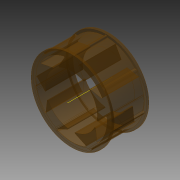
# Autodesk Inventor part: inner tread
Saved by Autodesk Inventor 2013 (Build 170138000, 138)
## iProperties
Created: 2013-05-09
Part Number: inner tread
Material: Generic
Document SubType Name: Modeling
Designer: grtstudent
Density: 1 g/cm^3
Author: grtstudent
Autodesk Inventor part; units mm, degrees
ref_plane "YZ Plane" through (0, 0, 0) normal (1, 0, 0) x (0, 1, 0)
ref_plane "XZ Plane" through (0, 0, 0) normal (0, 1, 0) x (-1, 0, 0)
ref_plane "XY Plane" through (0, 0, 0) normal (0, 0, 1) x (1, 0, 0)
sketch "Sketch1" plane through (0, 0, 0) normal (0, 0, 1) x (1, 0, 0)
  circle A0 centre (0, 0) radius 44.45
  circle A1 centre (11.1973, -15.4118) radius 1.905
  circle A2 centre (-18.1176, 5.8868) radius 1.905
  circle A3 centre (0, 19.05) radius 1.905
  circle A4 centre (-11.1973, -15.4118) radius 1.905
  circle A5 centre (18.1176, 5.8868) radius 1.905
  line L0 (-6.4158, 0) -> (-3.2079, 5.5563)
  line L1 (-3.2079, 5.5563) -> (3.2079, 5.5563)
  line L2 (3.2079, 5.5563) -> (6.4158, 0)
  line L3 (6.4158, 0) -> (3.2079, -5.5563)
  line L4 (3.2079, -5.5563) -> (-3.2079, -5.5563)
  line L5 (-3.2079, -5.5563) -> (-6.4158, 0)
  arc A6 (-6.9808, 33.2105) -> (-7.631, 34.0811) centre (-7.5009, 33.5002) ccw
  arc A7 (-7.631, 34.0811) -> (-30.055, 17.7891) centre (0, 0) ccw
  arc A8 (-30.055, 17.7891) -> (-29.4279, 16.9018) centre (-29.5427, 17.4859) ccw
  line L6 (-18.3896, 19.0716) -> (-29.4279, 16.9018)
  arc A9 (-17.8563, 18.0641) -> (-18.3896, 19.0716) centre (-18.2748, 18.4875) ccw
  arc A10 (-17.8563, 18.0641) -> (-25.0639, -4.1185) centre (0, 0) ccw
  arc A11 (-26.0876, -4.6201) -> (-25.0639, -4.1185) centre (-25.6513, -4.215) ccw
  line L7 (-33.7423, 3.6235) -> (-26.0876, -4.6201)
  arc A12 (-33.7423, 3.6235) -> (-34.7712, 3.2742) centre (-34.1785, 3.2184) ccw
  arc A13 (-34.7712, 3.2742) -> (-26.206, -23.0869) centre (0, 0) ccw
  arc A14 (-26.206, -23.0869) -> (-25.1682, -22.7646) centre (-25.7593, -22.6933) ccw
  line L8 (-23.8209, -11.5961) -> (-25.1682, -22.7646)
  arc A15 (-22.6979, -11.4002) -> (-23.8209, -11.5961) centre (-23.2299, -11.6674) ccw
  arc A16 (-22.6979, -11.4002) -> (-3.8282, -25.1098) centre (0, 0) ccw
  arc A17 (-3.6675, -26.2384) -> (-3.8282, -25.1098) centre (-3.918, -25.6984) ccw
  line L9 (-13.873, -30.9711) -> (-3.6675, -26.2384)
  arc A18 (-13.873, -30.9711) -> (-13.8588, -32.0576) centre (-13.6226, -31.5111) ccw
  arc A19 (-13.8588, -32.0576) -> (13.8588, -32.0576) centre (0, 0) ccw
  arc A20 (13.8588, -32.0576) -> (13.873, -30.9711) centre (13.6226, -31.5111) ccw
  line L10 (3.6675, -26.2384) -> (13.873, -30.9711)
  arc A21 (3.8282, -25.1098) -> (3.6675, -26.2384) centre (3.918, -25.6984) ccw
  arc A22 (3.8282, -25.1098) -> (22.6979, -11.4002) centre (0, 0) ccw
  arc A23 (23.8209, -11.5961) -> (22.6979, -11.4002) centre (23.2299, -11.6674) ccw
  line L11 (25.1682, -22.7646) -> (23.8209, -11.5961)
  arc A24 (25.1682, -22.7646) -> (26.206, -23.0869) centre (25.7593, -22.6933) ccw
  arc A25 (26.206, -23.0869) -> (34.7712, 3.2742) centre (0, 0) ccw
  arc A26 (34.7712, 3.2742) -> (33.7423, 3.6235) centre (34.1785, 3.2184) ccw
  line L12 (26.0876, -4.6201) -> (33.7423, 3.6235)
  arc A27 (25.0639, -4.1185) -> (26.0876, -4.6201) centre (25.6513, -4.215) ccw
  arc A28 (25.0639, -4.1185) -> (17.8563, 18.0641) centre (0, 0) ccw
  arc A29 (18.3896, 19.0716) -> (17.8563, 18.0641) centre (18.2748, 18.4875) ccw
  line L13 (29.4279, 16.9018) -> (18.3896, 19.0716)
  arc A30 (29.4279, 16.9018) -> (30.055, 17.7891) centre (29.5427, 17.4859) ccw
  arc A31 (30.055, 17.7891) -> (7.631, 34.0811) centre (0, 0) ccw
  arc A32 (7.631, 34.0811) -> (6.9808, 33.2105) centre (7.5009, 33.5002) ccw
  line L14 (12.4555, 23.383) -> (6.9808, 33.2105)
  arc A33 (11.6621, 22.5645) -> (12.4555, 23.383) centre (11.9354, 23.0933) ccw
  arc A34 (11.6621, 22.5645) -> (-11.6621, 22.5645) centre (0, 0) ccw
  arc A35 (-12.4555, 23.383) -> (-11.6621, 22.5645) centre (-11.9354, 23.0933) ccw
  line L15 (-6.9808, 33.2105) -> (-12.4555, 23.383)
  circle A36 centre (0, 0) radius 39.6875
  point P0 (-9.7181, 28.2968)
  point P1 (-23.3322, -11.081)
  dimension "d0" = 88.9
  dimension "d2" = 4.7625
  constraints: 61 point on circle, 37 centre point, 32 end point, 2 coincident, 1 midpoint, 42 other
  measures "d0" diameter of A0
  measures "d2" radial gap between concentric circles of A7 A36
extrude "Extrusion1" add sketch "Sketch1" along normal blind 36.5125 contours A36
sketch "Sketch2" plane through (0, 0, 0) normal (1, 0, 0) x (0, 1, 0)
  line L0 (-39.78, 34.1313) -> (-37.3062, 34.1313)
  line L1 (-37.3062, 34.1313) -> (-37.3062, 2.3813)
  line L2 (-37.3062, 2.3813) -> (-39.6875, 2.3813)
  line L3 (-39.6875, 0) -> (-39.6875, 36.5125) projected
  line L4 (0, 0) -> (0, 43.4091)
  dimension "d5" = 2.3813
  dimension "d6" = 2.3813
  dimension "d7" = 2.3813
  constraints: 8 end point, 2 parallel, 1 horizontal, 1 perpendicular, 1 point on line
  measures "d5" distance between parallel lines of L3 L1
  measures "d6" distance from line of L3.end L0
  measures "d7" distance from line of L3.start L2
revolve "Revolution1" cut sketch "Sketch2" angle 360 about axis through (0, 0, 0) along (0, 0, 1) fills toward (-38.5431, 34.0813) open curves L0 L1 L2
sketch "Sketch3" plane through (0, 0, 2.3813) normal (0, 0, 1) x (1, 0, 0)
  circle A0 centre (0, 0) radius 37.3062 projected
  line L0 (-1.1906, 37.2872) -> (1.1906, 37.2872)
  line L1 (1.1906, 38.0483) -> (1.1906, 38.081)
  line L2 (0.3969, 38.8747) -> (-0.3969, 38.8747)
  line L3 (-1.1906, 38.081) -> (-1.1906, 38.0483)
  line L4 (0, 0) -> (0, 39.6875)
  arc A1 (-0.3969, 38.8747) -> (-1.1906, 38.081) centre (-0.3969, 38.081) ccw
  arc A2 (1.1906, 38.081) -> (0.3969, 38.8747) centre (0.3969, 38.081) ccw
  arc A3 (-1.943, 37.2556) -> (-4.1916, 37.07) centre (0, 0) ccw
  arc A4 (-1.943, 37.2556) -> (-1.1906, 38.0483) centre (-1.9844, 38.0483) ccw
  arc A5 (2.6559, 37.2116) -> (1.943, 37.2556) centre (0, 0) ccw
  arc A6 (1.1906, 38.0483) -> (1.943, 37.2556) centre (1.9844, 38.0483) ccw
  arc A7 (1.943, 37.2556) -> (-1.943, 37.2556) centre (0, 0) ccw
  dimension "d10" = 2.3813
  dimension "d15" = 1.5875
  dimension "d16" = 0.7937
  dimension "d17" = 0.7937
  dimension "d18" = 0.7937
  constraints: 18 point on circle, 10 end point, 8 tangent, 7 centre point, 3 coincident, 3 equal radius, 2 parallel, 2 point on line, 1 horizontal, 1 perpendicular, 1 other
  measures "d10" distance between parallel lines of L1 L3
  measures "d15" distance between parallel lines of L0 L2
  measures "d16" radius of A1
  measures "d17" radius of A4
  measures "d18" radius of A6
extrude "Extrusion2" add sketch "Sketch3" along normal up to surface (31.75 mm away) contours A0 L4 L2 A2 L1 A6 | A4 L3 A1 L2 L4 A0
pattern_circular "Circular Pattern1" count 7 over 360 about axis through (0, 0, 18.2563) along (0, 0, -1) of "Extrusion2"
equation "\"d6\" = d5"
equation "\"d7\" = d6"
body "Solid1"
